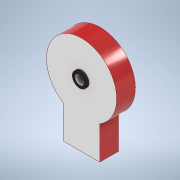
# Autodesk Inventor part: BigCounterWeight
Saved by Autodesk Inventor 2022 (Build 260153000, 153)
## iProperties
Created: 2021-04-24
Part Number: BigCounterWeight
Material: Generic
Document SubType Name: Modeling
Designer: Mick Veldhuis
Density: 1 g/cm^3
Appearance: Rubber - Black
Author: Mick Veldhuis
Autodesk Inventor part; units mm, degrees
ref_plane "YZ Plane" through (0, 0, 0) normal (1, 0, 0) x (0, 1, 0)
ref_plane "XZ Plane" through (0, 0, 0) normal (0, 1, 0) x (-1, 0, 0)
ref_plane "XY Plane" through (0, 0, 0) normal (0, 0, 1) x (1, 0, 0)
sketch "Sketch1" plane through (0, 0, 0) normal (0, 0, 1) x (1, 0, 0)
  arc A0 (78, -128.1249) -> (-78, -128.1249) centre (0, 0) ccw
  line L0 (78, -128.1249) -> (78, -270)
  line L1 (78, -270) -> (-78, -270)
  line L2 (-78, -270) -> (-78, -128.1249)
  line L3 (-78, -30) -> (78, -270) construction
  line L4 (78, -30) -> (-78, -270) construction
  constraints: 10 end point, 2 point on circle, 1 centre point, 1 coincident, 1 parallel
extrude "Extrusion1" add sketch "Sketch1" along normal blind 80
sketch "Sketch2" plane through (0, 0, 80) normal (0, 0, 1) x (1, 0, 0)
  circle A0 centre (0, 0) radius 20
  constraints: 1 centre point, 1 coincident
extrude "Extrusion2" cut sketch "Sketch2" against normal through all
sketch "Sketch3" plane through (0, 0, 80) normal (0, 0, 1) x (1, 0, 0)
  circle A0 centre (0, 0) radius 32
  constraints: 1 centre point, 1 coincident
sketch "Sketch4" plane through (0, 0, 80) normal (0, 0, 1) x (1, 0, 0)
  circle A0 centre (0, 0) radius 20
  constraints: 1 centre point, 1 coincident
extrude "Extrusion3" add sketch "Sketch3" along normal blind 8
extrude "Extrusion4" cut sketch "Sketch4" along normal blind 8
body "Solid1"
